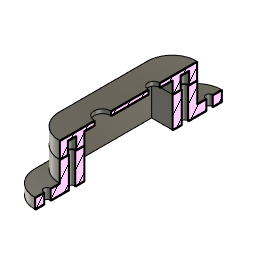
power-knob (Autodesk Fusion 360 design; units mm, degrees)
Autodesk Fusion 360 part; units mm, degrees
sketch "Skizze2" plane through (0, 0, 0) normal (0, 0, 1) x (1, 0, 0)
  line L0 (12, 33.5) -> (-12, 33.5)
  line L1 (-12, 33.5) -> (-12, -33.5)
  line L2 (-12, -33.5) -> (12, -33.5)
  line L3 (12, -33.5) -> (12, 33.5)
  line L4 (12, 33.5) -> (-12, -33.5) construction
  line L5 (-12, 33.5) -> (12, -33.5) construction
  circle A0 centre (0, -12.5) radius 4
  circle A1 centre (0, 12.5) radius 2.75
  circle A2 centre (0, 27.5) radius 2.1
  circle A3 centre (0, 39.5) radius 1.6
  circle A4 centre (0, -27.5) radius 2.1
  line L6 (-12, 21.5) -> (12, 21.5)
  line L7 (12, 21.5) -> (12, 45.5)
  line L8 (12, 45.5) -> (-12, 45.5)
  line L9 (-12, 45.5) -> (-12, 21.5)
  circle A5 centre (0, -39.5) radius 1.6
  line L10 (-12, -21.5) -> (12, -21.5)
  line L11 (12, -21.5) -> (12, -45.5)
  line L12 (12, -45.5) -> (-12, -45.5)
  line L13 (-12, -45.5) -> (-12, -21.5)
  circle A6 centre (0, 33.5) radius 12
  circle A7 centre (0, 21.5) radius 12
  circle A8 centre (0, -33.5) radius 12
  circle A9 centre (0, -21.5) radius 12
  line L14 (-10, 31.5) -> (-10, -31.5)
  line L15 (-10, -31.5) -> (10, -31.5)
  line L16 (10, -31.5) -> (10, 31.5)
  line L17 (10, 31.5) -> (-10, 31.5)
  circle A10 centre (0, 27.5) radius 1.6
  circle A11 centre (0, -27.5) radius 1.6
  dimension "d15" = 24
  dimension "d16" = 8
  dimension "d17" = 5.5
  dimension "d18" = 4.2
  dimension "d19" = 3.2
  dimension "d20" = 6
  dimension "d21" = 15
  dimension "d22" = 4.2
  dimension "d23" = 6
  dimension "d24" = 15
  dimension "d25" = 25
  dimension "d26" = 12
  dimension "d27" = 6
  dimension "d28" = 6
  dimension "d29" = 3.2
  dimension "d30" = 6
  dimension "d31" = 12
  dimension "d32" = 6
  dimension "d36" = 24
  dimension "d37" = 24
  dimension "d38" = -2
  dimension "d48" = 3.2
  dimension "d49" = 3.2
  constraint horizontal L0
  constraint perpendicular L0 L1
  constraint parallel L0 L2
  constraint parallel L1 L3
  constraint coincident L4 origin
  constraint coincident L5 origin
  constraint vertical origin A1.centre
  constraint vertical origin A2.centre
  constraint vertical origin A0.centre
  constraint vertical origin A4.centre
  constraint vertical origin A3.centre
  constraint horizontal L6
  constraint vertical L7
  constraint horizontal L8
  constraint vertical L9
  constraint coincident L1 L6.start
  constraint horizontal L10
  constraint vertical L11
  constraint horizontal L12
  constraint vertical L13
  constraint coincident L1 L10.start
  constraint tangent L8 A6
  constraint tangent L9 A6
  constraint tangent L7 A6
  constraint tangent L0 A7
  constraint tangent L1 A7
  constraint tangent L3 A7
  constraint tangent L12 A8
  constraint tangent L13 A8
  constraint tangent L11 A8
  constraint tangent L2 A9
  constraint tangent L1 A9
  constraint tangent L3 A9
  constraint vertical origin A5.centre
  constraint concentric A2 A10
  constraint concentric A4 A11
  measures "d15" distance of L1.end L2.end
  measures "d16" diameter of A0
  measures "d17" diameter of A1
  measures "d18" diameter of A2
  measures "d19" diameter of A3
  measures "d20" distance of L0 A2.centre
  measures "d21" distance of A1.centre A2.centre
  measures "d22" diameter of A4
  measures "d23" distance of L2 A4.centre
  measures "d24" distance of A0.centre A4.centre
  measures "d25" distance of A0.centre A1.centre
  measures "d26" distance of A2.centre A3.centre
  measures "d27" distance of A2.centre L6
  measures "d28" distance of A3.centre L8
  measures "d29" diameter of A5
  measures "d30" distance of A4.centre L10
  measures "d31" distance of A4.centre A5.centre
  measures "d32" distance of A5.centre L12
  measures "d36" distance of L10.start L10.end
  measures "d37" distance of L6.start L6.end
  measures "d48" diameter of A10
  measures "d49" diameter of A11
extrude "Extrusion3" add sketch "Skizze2" along normal blind 5 contours L0 A6 A7 L16 L17 | L0 A6 | L3 L7 A6 A7 | L0 A6 A7 L14 L17 | A7 L17 | L6 A7 L16 | L6 A6 A7 L16 | L3 A7 A9 L16 | A6 A7 L16 | L1 L9 A6 A7 | A7 L16 L17 | A6 A7 L14 L16 L17 | A7 L14 L17 | L10 A8 A9 L16 | L10 A9 L16 | L3 L11 A8 A9 | L6 A6 L16 | L1 A7 A9 L14 | L6 A6 A7 L14 | L6 A7 L14 | A6 A7 L14 | L2 A8 | L2 A8 A9 L15 L16 | L10 A8 L16 | A8 A9 L16 | L6 A6 L14 | L1 L13 A8 A9 | L10 A9 L14 | L10 A8 A9 L14 | L2 A8 A9 L14 L15 | A9 L15 | L10 A8 L14 | A8 A9 L14 L15 L16 | A9 L15 L16 | A8 A9 L14 | A9 L14 L15 makes body 1
sketch "Skizze5" plane through (0, 0, 5) normal (0, 0, 1) x (-1, 0, 0)
  circle A0 centre (0, -39.5) radius 1.6
  circle A1 centre (0, 39.5) radius 1.6
  circle A2 centre (0, 27.5) radius 2.1
  circle A3 centre (0, -27.5) radius 2.1
  line L0 (10, 21.5) -> (10, -21.5)
  line L1 (10, -21.5) -> (-10, -21.5)
  line L2 (-10, -21.5) -> (-10, 21.5)
  line L3 (-10, 21.5) -> (10, 21.5)
  line L4 (-12, 33.5) -> (-12, -33.5)
  arc A4 (-12, -33.5) -> (12, -33.5) centre (0, -33.5) ccw
  line L5 (12, -33.5) -> (12, 33.5)
  arc A5 (12, 33.5) -> (-12, 33.5) centre (0, 33.5) ccw
  circle A6 centre (0, -21.5) radius 12
  line L6 (12, -21.5) -> (-12, -21.5)
  line L7 (10, -31.5) -> (10, 31.5)
  line L8 (-10, 31.5) -> (-10, -31.5)
  line L9 (-12, 33.5) -> (-12, -33.5)
  circle A7 centre (0, 21.5) radius 12
  circle A8 centre (0, -27.5) radius 2.1
  circle A9 centre (0, 27.5) radius 2.1
  line L10 (12, -33.5) -> (12, 33.5)
  line L11 (12, 21.5) -> (-12, 21.5)
extrude "Extrusion4" add sketch "Skizze5" along normal blind 18 contours L0 L7 A7 L11 | L3 L7 L8 A7 L11 | L7 A7 L11 | L0 L5 A6 L7 A7 L10 | L8 A7 L11 | L2 L8 A7 L11 | L0 A6 L6 L7 | L2 L4 A6 L8 L9 A7 | A6 L6 L7 | L1 A6 L6 L7 L8 | L2 A6 L6 L8 | A6 L6 L8 bodies 1
sketch "Skizze6" plane through (0, 0, 23) normal (0, 0, 1) x (-1, 0, 0)
  line L0 (10, 21.5) -> (10, -21.5)
  line L1 (10, -21.5) -> (-10, -21.5)
  line L2 (-10, -21.5) -> (-10, 21.5)
  line L3 (-10, 21.5) -> (10, 21.5)
  circle A0 centre (0, 27.5) radius 2.1
  circle A1 centre (0, -27.5) radius 2.1
  arc A2 (-12, -21.5) -> (12, -21.5) centre (0, -21.5) ccw
  line L4 (12, -21.5) -> (12, 21.5)
  arc A3 (12, 21.5) -> (-12, 21.5) centre (0, 21.5) ccw
  line L5 (-12, 21.5) -> (-12, -21.5)
  circle A4 centre (0, -12.5) radius 2.75
  circle A5 centre (0, 12.5) radius 4
extrude "Extrusion5" add sketch "Skizze6" against normal blind 2 contours L0 L1 L2 L3 | A0 | A1 bodies 1
ref_plane "Arbeitsebene1" through (0, 0, 15) normal (0, 0, 1) x (-1, 0, 0)
split "Teilen1" by plane through (0, 0, 15) normal (0, 0, 1) bodies 1 makes body 2 at (9.2013, -3.5882, 23)
ref_plane "Arbeitsebene2" through (0, 0, 11.5) normal (1, 0, 0) x (0, 1, 0)
extrude "Extrusion6" add sketch "Skizze2" along normal up to surface (15 mm away) contours A2 | A4 bodies 1
equation "d22 = d18"
equation "d23 = d20"
equation "d24 = d21"
equation "d27 = d20"
equation "d28 = d26 - d20"
equation "d29 = d19"
equation "d30 = d20"
equation "d31 = d26"
equation "d32 = d28"
equation "d36 = d15"
equation "d37 = d15"
equation "d48 = d19"
equation "d49 = d19"
